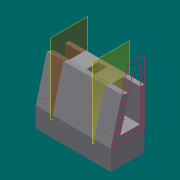
# Autodesk Inventor part: 知能ロボコン土台1.1
Saved by Autodesk Inventor 2013 (Build 170138000, 138)
## iProperties
Created: 2014-08-06
Part Number: 知能ロボコン土台1.1
Material: 一般
Document SubType Name: Modeling
Designer: horumo136
Density: 1 g/cm^3
Author: horumo136
Autodesk Inventor part; units mm, degrees
ref_plane "YZ Plane" through (0, 0, 0) normal (1, 0, 0) x (0, 1, 0)
ref_plane "XZ Plane" through (0, 0, 0) normal (0, 1, 0) x (-1, 0, 0)
ref_plane "XY Plane" through (0, 0, 0) normal (0, 0, 1) x (1, 0, 0)
sketch "スケッチ1" plane through (0, 0, 0) normal (1, 0, 0) x (0, 1, 0)
  line L0 (0, 0) -> (20.7055, 77.2741)
  line L1 (0, 0) -> (80, 0) construction
  line L2 (20.7055, 77.2741) -> (20.7055, 0)
  line L3 (20.7055, 0) -> (0, 0)
  line L4 (0, 0) -> (20.7055, 0)
  line L5 (0, 0) -> (40, 0)
  line L6 (40, 0) -> (40, 77.2741)
  line L7 (40, 77.2741) -> (20.7055, 77.2741)
  dimension "d0" = 80
  dimension "d1" = 75
  dimension "d2" = 15
  dimension "d44" = 40
  constraints: 16 end point, 2 perpendicular, 1 equal length, 1 horizontal, 1 midpoint, 1 parallel
  measures "d0" distance of L0.start L0.end
  measures "d1" angle of L1 L0
  measures "d2" angle of L0 L2
  measures "d44" distance of L0.start L5.end
extrude "押し出し1" add sketch "スケッチ1" along normal blind 90
sketch "スケッチ2" plane through (0, 0, 0) normal (0, -0.9659258, 0.258819) x (1, 0, 0)
  line L0 (0, 80) -> (10, 80)
  line L1 (10, 80) -> (10, 70)
  line L2 (10, 70) -> (0, 70)
  line L3 (0, 70) -> (0, 80)
  line L4 (90, 80) -> (80, 80)
  line L5 (80, 80) -> (80, 70)
  line L6 (80, 70) -> (90, 70)
  line L7 (90, 70) -> (90, 80)
  line L8 (90, 0) -> (80, 0)
  line L9 (80, 0) -> (80, 10)
  line L10 (80, 10) -> (90, 10)
  line L11 (90, 10) -> (90, 0)
  line L12 (0, 0) -> (10, 0)
  line L13 (10, 0) -> (10, 10)
  line L14 (10, 10) -> (0, 10)
  line L15 (0, 10) -> (0, 0)
  dimension "d5" = 10
  dimension "d6" = 10
  dimension "d7" = 10
  dimension "d8" = 10
  dimension "d9" = 10
  dimension "d10" = 10
  dimension "d11" = 10
  dimension "d12" = 10
  constraints: 32 end point, 8 parallel, 4 coincident, 4 horizontal, 4 perpendicular
  measures "d5" distance of L1.end L2.end
  measures "d6" distance of L0.end L1.end
  measures "d7" distance of L6.end L5.end
  measures "d8" distance of L5.end L4.end
  measures "d9" distance of L9.end L10.end
  measures "d10" distance of L8.end L9.end
  measures "d11" distance of L14.end L13.end
  measures "d12" distance of L13.end L12.end
hole "穴1" at (10, 18.1173, 67.6148) at (10, 2.5882, 9.6593) at (80, 2.5882, 9.6593) at (80, 18.1173, 67.6148) direction (0, 0.9659258, -0.258819) diameter 2.5 depth 20 tip angle 118
sketch "スケッチ4" plane through (90, 0, 0) normal (1, 0, 0) x (0, 0, -1)
  line L0 (-77.2741, 20.7055) -> (0, 0) projected
  line L1 (0, 0) -> (0, 20.7055) projected
  line L2 (-8, 20.7055) -> (-8, 2.1436)
  line L3 (0, 12.7055) -> (-47.4177, 12.7055)
  line L4 (-46.3644, 20.7055) -> (0, 8.2822)
  line L5 (-77.2741, 40) -> (-77.2741, 20.7055) projected
  line L6 (-46.3644, 20.7055) -> (-69.8423, 26.9964)
  line L7 (-69.8423, 26.9964) -> (-69.8423, 34.9964)
  line L8 (-69.8423, 34.9964) -> (-8, 34.9964)
  line L9 (-8, 34.9964) -> (-8, 20)
  point P0 (-16.508, 12.7055)
  point P1 (-8, 12.7055)
  point P2 (-8, 10.4258)
  dimension "d34" = 8
  dimension "d36" = 8
  dimension "d45" = 8
  constraints: 14 end point, 11 point on line, 2 parallel, 1 collinear, 1 perpendicular
  measures "d34" distance between parallel lines of L1 L2
  measures "d36" distance between parallel lines of L0 L4
  measures "d45" distance of L6.end L7.end
ref_plane "作業平面1" through (45, 0, 0) normal (-1, 0, 0) x (0, 0, 1)
extrude "押し出し4" cut sketch "スケッチ4" against normal blind 45 contours L4 L6 L7 L8 L9 L2 L3 | L3 L2 L4
mirror "ミラー1" about plane through (45, 0, 0) normal (-1, 0, 0) of "押し出し4"
sketch "スケッチ6" plane through (0, 0, 0) normal (0, 0, -1) x (-1, 0, 0)
  line L0 (-90, 40) -> (-75, 40)
  line L1 (-75, 40) -> (-75, 30)
  line L2 (-75, 30) -> (-90, 30)
  line L3 (-90, 30) -> (-90, 40)
  line L4 (-90, 0) -> (-75, 0)
  line L5 (-75, 0) -> (-75, 10)
  line L6 (-75, 10) -> (-90, 10)
  line L7 (-90, 10) -> (-90, 0)
  line L8 (0, 40) -> (-15, 40)
  line L9 (-15, 40) -> (-15, 30)
  line L10 (-15, 30) -> (0, 30)
  line L11 (0, 30) -> (0, 40)
  line L12 (0, 0) -> (-15, 0)
  line L13 (-15, 0) -> (-15, 10)
  line L14 (-15, 10) -> (0, 10)
  line L15 (0, 10) -> (0, 0)
  point P0 (-45, 30)
  point P1 (-45, 10)
  dimension "d49" = 15
  dimension "d50" = 10
  dimension "d51" = 10
  dimension "d52" = 15
  dimension "d53" = 10
  dimension "d54" = 10
  constraints: 32 end point, 8 parallel, 7 coincident, 4 horizontal, 4 perpendicular
  measures "d49" distance of L1.end L2.end
  measures "d50" distance of L0.end L1.end
  measures "d51" distance of L5.end L4.end
  measures "d52" distance of L10.end L9.end
  measures "d53" distance of L9.end L8.end
  measures "d54" distance of L12.end L13.end
hole "穴3" at (45, 30, 0) at (45, 10, 0) at (15, 10, 0) at (15, 30, 0) at (75, 30, 0) at (75, 10, 0) direction (0, 0, 1) diameter 2.5 depth 8 tip angle 118
sketch "スケッチ7" plane through (90, 0, 0) normal (1, 0, 0) x (0, 0, -1)
  line L0 (-69.8423, 34.9964) -> (-8, 34.9964) projected
  line L1 (-8, 34.9964) -> (-8, 10.4258) projected
  line L2 (-8, 10.4258) -> (-69.8423, 26.9964) projected
  line L3 (-69.8423, 26.9964) -> (-69.8423, 34.9964) projected
  line L4 (0, 0) -> (0, 40) projected
  line L5 (0, 40) -> (-77.2741, 40) projected
  line L6 (-77.2741, 40) -> (-77.2741, 20.7055) projected
  line L7 (-77.2741, 20.7055) -> (0, 0) projected
ref_plane "作業平面2" through (70, 0, 0) normal (1, 0, 0) x (0, 0, -1)
sketch "スケッチ8" plane through (70, 0, 0) normal (1, 0, 0) x (0, 0, -1)
  line L0 (-5.9326, 37.4868) -> (-71.6084, 37.4868)
  line L1 (-71.6084, 37.4868) -> (-71.6084, 19.3326)
  line L2 (-28.0915, 7.5857) -> (-5.9326, 7.5857)
  line L3 (-5.9326, 7.5857) -> (-5.9326, 37.4868)
  line L4 (-28.0915, 7.5857) -> (-71.6084, 19.3326)
  point P0 (0, 0)
  constraints: 10 end point, 2 parallel, 1 horizontal, 1 perpendicular
extrude "押し出し5" add sketch "スケッチ8" against normal blind 20
ref_plane "作業平面3" through (20, 0, 0) normal (-1, 0, 0) x (0, 0, 1)
sketch "スケッチ9" plane through (20, 0, 0) normal (-1, 0, 0) x (0, 0, 1)
  line L0 (5.473, 36.709) -> (72.4836, 36.709)
  line L1 (72.4836, 36.709) -> (72.4836, 22.6929)
  line L2 (20.9575, 8.6767) -> (5.473, 8.6767)
  line L3 (5.473, 8.6767) -> (5.473, 36.709)
  line L4 (20.9575, 8.6767) -> (72.4836, 22.6929)
  point P0 (0, 0)
  constraints: 10 end point, 2 parallel, 1 horizontal, 1 perpendicular
extrude "押し出し6" add sketch "スケッチ9" against normal blind 20
sketch "スケッチ10" plane through (0, 0, 0) normal (-1, 0, 0) x (0, 0, 1)
  line L0 (77.2741, 40) -> (47.2741, 40)
  line L1 (50.1134, 10.3528) -> (77.2741, 10.3528)
  line L2 (77.2741, 10.3528) -> (77.2741, 40)
  line L3 (69.8423, 26.9964) -> (8, 10.4258) projected
  line L4 (77.2741, 20.7055) -> (0, 0) projected
  line L5 (47.2741, 20.9493) -> (49.3446, 13.2219)
  line L6 (49.3446, 13.2219) -> (50.1134, 10.3528)
  line L7 (47.2741, 40) -> (47.2741, 20.9493)
  line L8 (47.2741, 12.667) -> (47.2741, 10.3528)
  dimension "d68" = 30
  constraints: 14 end point, 3 parallel, 3 perpendicular, 3 point on line, 1 collinear, 1 horizontal
  measures "d68" distance of L1.end L8.end
extrude "押し出し7" cut sketch "スケッチ10" against normal blind 100
sketch "スケッチ11" plane through (0, 0, 0) normal (0, 0, -1) x (-1, 0, 0)
  circle A0 centre (-75, 30) radius 1.25 projected
  circle A1 centre (-15, 10) radius 1.25 projected
  circle A2 centre (-45, 30) radius 1.25 projected
  circle A3 centre (-45, 10) radius 1.25 projected
  circle A4 centre (-15, 30) radius 1.25 projected
  circle A5 centre (-75, 10) radius 1.25 projected
  line L0 (0, 0) -> (0, 40) projected
  line L1 (0, 40) -> (-90, 40) projected
  line L2 (-90, 0) -> (-90, 40) projected
  line L3 (0, 0) -> (-90, 0) projected
extrude "押し出し8" add sketch "スケッチ11" along normal blind 24
sketch "スケッチ12" plane through (0, 0, -24) normal (0, 0, -1) x (-1, 0, 0)
  circle A0 centre (-75, 10) radius 1.25 projected
  circle A1 centre (-45, 10) radius 1.25 projected
  circle A2 centre (-15, 10) radius 1.25 projected
extrude "押し出し9" cut sketch "スケッチ12" against normal blind 37
